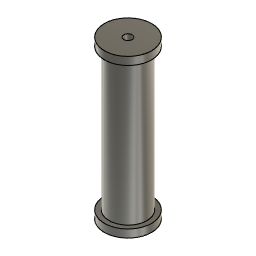
Luka (Autodesk Fusion 360 design; units mm, degrees)
Autodesk Fusion 360 part; units mm, degrees
sketch "Sketch1" plane through (0, 0, 0) normal (0, 0, 1) x (1, 0, 0)
  circle A0 centre (50, 25) radius 15
  dimension "d1" = 30
  measures "d1" diameter of A0
extrude "Extrude1" add sketch "Sketch1" along normal blind 60
sketch "Sketch2" plane through (0, 0, 60) normal (0, 0, 1) x (-1, 0, 0)
  circle A0 centre (-50, -25) radius 15
  circle A1 centre (-50, -25) radius 2.5
  dimension "d4" = 5
  constraint concentric A0 A1
  measures "d4" diameter of A1
extrude "Extrude2" cut sketch "Sketch2" against normal blind 55 contours A1
sketch "Sketch3" plane through (0, 0, 60) normal (0, 0, 1) x (-1, 0, 0)
  circle A0 centre (-50, -25) radius 2.5
  circle A1 centre (-50, -25) radius 15
  circle A2 centre (-50, -25) radius 12
  dimension "d7" = 24
  constraint concentric A0 A2
  measures "d7" diameter of A2
extrude "Extrude3" cut sketch "Sketch3" against normal blind 55 contours A1
sketch "Sketch4" plane through (0, 0, 60) normal (0, 0, 1) x (-1, 0, 0)
  circle A0 centre (-50, -25) radius 12
  circle A1 centre (-50, -25) radius 2.5
  circle A2 centre (-50, -25) radius 15
  dimension "d10" = 30
  constraint concentric A0 A2
  measures "d10" diameter of A2
extrude "Extrude4" add sketch "Sketch4" against normal blind 5 contours A2
extrude "Extrude5" cut 1 faces at (63.9442, 25.7452, 5) along direction (0, 0, 1) blind 55
extrude "Extrude6" add 1 faces at (41.2207, 25.7204, 60) along direction (0, 0, -1) blind 55
extrude "Extrude7" add 1 faces at (41.2207, 25.7204, 60) along direction (0, 0, 1) blind 35
sketch "Sketch5" plane through (0, 0, 95) normal (0, 0, 1) x (-1, 0, 0)
  circle A0 centre (-50, -25) radius 12
  circle A1 centre (-50, -25) radius 2.5
  circle A2 centre (-50, -25) radius 2.65
  dimension "d19" = 5.3
  constraint concentric A0 A2
  measures "d19" diameter of A2
extrude "Extrude8" cut sketch "Sketch5" against normal blind 90 contours A2
sketch "Sketch6" plane through (0, 0, 95) normal (0, 0, 1) x (-1, 0, 0)
  circle A0 centre (-50, -25) radius 2.65
  circle A1 centre (-50, -25) radius 12
  circle A2 centre (-50, -25) radius 15
  dimension "d22" = 30
  constraint concentric A0 A2
  measures "d22" diameter of A2
extrude "Extrude9" add sketch "Sketch6" along normal blind 5 contours A1 | A2
